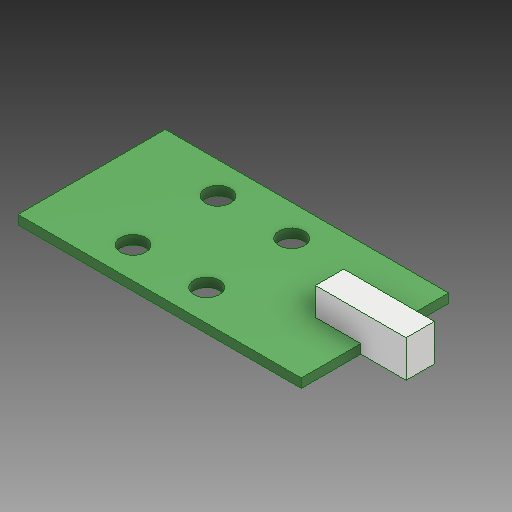
# Autodesk Inventor part: IGBT_Platine
Saved by Autodesk Inventor 2019 (Build 230136000, 136)
## iProperties
Created: 2018-04-27
Part Number: IGBT_Platine
Material: Generic
Document SubType Name: Modeling
Designer: Phil Erle
Density: 1 g/cm^3
Appearance: Smooth - Dark Forest Green
Author: Phil Erle
Autodesk Inventor part; units mm, degrees
ref_plane "YZ Plane" through (0, 0, 0) normal (1, 0, 0) x (0, 1, 0)
ref_plane "XZ Plane" through (0, 0, 0) normal (0, 1, 0) x (-1, 0, 0)
ref_plane "XY Plane" through (0, 0, 0) normal (0, 0, 1) x (1, 0, 0)
sketch "Sketch1" plane through (0, 0, 0) normal (0, 0, 1) x (1, 0, 0)
  line L0 (-25, -13) -> (25, -13)
  line L1 (25, -13) -> (25, 13)
  line L2 (25, 13) -> (-25, 13)
  line L3 (-25, 13) -> (-25, -13)
  line L4 (-25, -13) -> (25, 13) construction
  line L5 (25, -13) -> (-25, 13) construction
  point P0 (0, 0)
  dimension "d0" = 50
  dimension "d1" = 26
  constraints: 12 end point, 2 midpoint, 2 parallel, 1 horizontal, 1 perpendicular
  measures "d0" distance of L1.end L2.end
  measures "d1" distance of L2.end L0.start
extrude "Extrusion1" add sketch "Sketch1" along normal blind 1.6
sketch "Sketch2" plane through (0, 0, 1.6) normal (0, 0, 1) x (1, 0, 0)
  line L0 (-10.2, -7.5) -> (2.8, -7.5) construction
  line L1 (2.8, -7.5) -> (2.8, 7.5) construction
  line L2 (2.8, 7.5) -> (-10.2, 7.5) construction
  line L3 (-10.2, 7.5) -> (-10.2, -7.5) construction
  line L4 (-25, 13) -> (-25, -13) construction
  point P0 (0, 0)
  point P1 (2.8, 0)
  dimension "d4" = 13
  dimension "d5" = 15
  dimension "d6" = 14.8
  constraints: 8 end point, 4 coincident, 2 parallel, 1 horizontal, 1 horizontal alignment, 1 midpoint, 1 perpendicular
  measures "d4" distance of L1.end L2.end
  measures "d5" distance of L2.end L0.start
  measures "d6" distance from line of L2.end L4
hole "Hole1" at (-10.2, 7.5, 1.6) at (2.8, 7.5, 1.6) at (2.8, -7.5, 1.6) at (-10.2, -7.5, 1.6) direction (0, 0, -1) diameter 4.5 end through all clearance for "Countersunk Flat Head Screw DIN EN ISO 2009" size "M4" standard "DIN"
sketch "Sketch3" plane through (25, -13, 0) normal (1, 0, 0) x (0, 0, -1)
  line L0 (0, 10.5) -> (-6.5, 10.5)
  line L1 (-6.5, 10.5) -> (-6.5, 15.5)
  line L2 (-6.5, 15.5) -> (0, 15.5)
  line L3 (0, 15.5) -> (0, 10.5)
  line L4 (0, 0) -> (0, 26) projected
  point P0 (0, 13)
  point P1 (0, 13)
  point P2 (0, 13)
  point P3 (0, 13)
  dimension "d14" = 5
  dimension "d15" = 6.5
  constraints: 8 end point, 3 midpoint, 2 parallel, 1 coincident, 1 horizontal, 1 perpendicular, 1 vertical alignment
  measures "d14" distance of L0.end L1.end
  measures "d15" distance of L1.end L2.end
extrude "Extrusion2" add sketch "Sketch3" along normal mid plane 16
body "Solid1"
